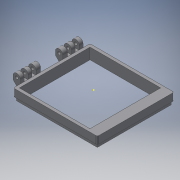
# Autodesk Inventor part: tampa extra
Saved by Autodesk Inventor 2019.4 (Build 234330000, 330)
## iProperties
Created: 2019-11-08
Part Number: tampa extra
Material: Genérico
Document SubType Name: Modeling
Designer: natha
Density: 1 g/cm^3
Appearance: Padrão
Author: natha
Autodesk Inventor part; units mm, degrees
ref_plane "YZ Plane" through (0, 0, 0) normal (1, 0, 0) x (0, 1, 0)
ref_plane "XZ Plane" through (0, 0, 0) normal (0, 1, 0) x (-1, 0, 0)
ref_plane "XY Plane" through (0, 0, 0) normal (0, 0, 1) x (1, 0, 0)
sketch "Esboço3" plane through (0, 0, 0) normal (0, 1, 0) x (-1, 0, 0)
  line L0 (-57, 52) -> (57, 52)
  line L1 (57, 52) -> (57, -52)
  line L2 (57, -52) -> (-57, -52)
  line L3 (-57, -52) -> (-57, 52)
  line L4 (-57, 52) -> (57, -52) construction
  line L5 (57, 52) -> (-57, -52) construction
  line L6 (-53, 48) -> (53, 48)
  line L7 (53, 48) -> (53, -48)
  line L8 (53, -48) -> (-53, -48)
  line L9 (-53, -48) -> (-53, 48)
  line L10 (-53, 48) -> (53, -48) construction
  line L11 (53, 48) -> (-53, -48) construction
  point P0 (0, 0)
  dimension "d9" = 104
  dimension "d10" = 114
  dimension "d11" = 106
  dimension "d12" = 96
  constraints: 24 end point, 4 midpoint, 4 parallel, 2 horizontal, 2 perpendicular
  measures "d9" distance of L0.end L1.end
  measures "d10" distance of L1.end L2.end
  measures "d11" distance of L7.end L8.end
  measures "d12" distance of L8.end L6.start
extrude "Extrusão2" add sketch "Esboço3" along normal blind 10
sketch "Esboço4" plane through (0, 0, 0) normal (0, -1, 0) x (1, 0, 0)
  line L0 (-53, -48) -> (53, -48) projected
  line L1 (-53, 48) -> (53, 48)
  line L2 (53, 48) -> (53, -48)
  line L3 (53, -48) -> (-53, -48)
  line L4 (-53, -48) -> (-53, 48)
  line L5 (-53, 48) -> (53, -48) construction
  line L6 (53, 48) -> (-53, -48) construction
  line L7 (-55, 50) -> (55, 50)
  line L8 (55, 50) -> (55, -50)
  line L9 (55, -50) -> (-55, -50)
  line L10 (-55, -50) -> (-55, 50)
  line L11 (-55, 50) -> (55, -50) construction
  line L12 (55, 50) -> (-55, -50) construction
  point P0 (0, 0)
  dimension "d15" = 100
  dimension "d16" = 96
  dimension "d17" = 110
  dimension "d18" = 106
  constraints: 24 end point, 4 midpoint, 4 parallel, 2 horizontal, 2 perpendicular
  measures "d15" distance of L7.end L8.end
  measures "d16" distance of L1.end L0.end
  measures "d17" distance of L8.end L9.end
  measures "d18" distance of L0.start L0.end
extrude "Extrusão3" add sketch "Esboço4" along normal blind 5
sketch "Esboço5" plane through (0, 10, 0) normal (0, 1, 0) x (1, 0, 0)
  line L0 (53, 48) -> (53, -48) projected
  line L1 (53, -48) -> (43, -48)
  line L2 (43, -48) -> (43, 48)
  line L3 (43, 48) -> (53, 48)
  line L4 (53, 48) -> (53, -48)
  point P0 (0, 0)
  dimension "d21" = 10
  constraints: 8 end point, 2 parallel, 1 horizontal, 1 perpendicular
  measures "d21" distance of L0.end L1.end
extrude "Extrusão4" add sketch "Esboço5" against normal blind 2
sketch "Esboço6" plane through (0, 8, 0) normal (0, -1, 0) x (1, 0, 0)
  line L0 (43, 48) -> (43, -48) projected
  line L1 (43, 48) -> (45, 48)
  line L2 (45, 48) -> (45, -48)
  line L3 (45, -48) -> (43, -48)
  line L4 (43, -48) -> (43, 48)
  point P0 (0, 0)
  dimension "d24" = 2
  constraints: 8 end point, 2 parallel, 1 horizontal, 1 perpendicular
  measures "d24" distance of L2.end L3.end
extrude "Extrusão5" add sketch "Esboço6" along normal blind 13
sketch "Esboço7" plane through (0, 10, 0) normal (0, 1, 0) x (1, 0, 0)
  point P0 (0, 0)
sketch "Esboço9" plane through (-57, 0, 52) normal (0, 0, 1) x (1, 0, 0)
  line L0 (114, 0) -> (0, 0) projected
  line L1 (0, 0) -> (-9.4142, 9.4142)
  line L2 (0, 0) -> (0, 10) projected
  line L3 (0, 10) -> (-10, 10) construction
  line L4 (0, 10) -> (0, 15.06) construction
  line L5 (0, 15.06) -> (-10, 15.06) construction
  arc A0 (0, 15.06) -> (-10, 15.06) centre (-5, 15.06) ccw
  line L6 (-10, 10.8284) -> (-10, 15.06)
  line L7 (0, 15.06) -> (0, 0)
  circle A1 centre (-5, 15.06) radius 2
  arc A2 (-10, 10.8284) -> (-9.4142, 9.4142) centre (-8, 10.8284) ccw
  point P0 (57, 0)
  dimension "d29" = 45
  dimension "d30" = 5.06
  dimension "d31" = 4
  dimension "d32" = 2
  constraints: 12 end point, 4 point on circle, 3 centre point, 3 tangent, 2 point on line, 2 vertical, 1 coincident, 1 collinear, 1 horizontal, 1 midpoint, 1 perpendicular
  measures "d29" angle of L1 L2
  measures "d30" distance of L2.end L4.end
  measures "d31" diameter of A1
  measures "d32" radius of A2
extrude "Extrusão6" add sketch "Esboço9" against normal blind 104
sketch "Esboço10" plane through (-67, 10.8284, 52) normal (-1, 0, 0) x (0, 0, 1)
  line L0 (-52, -10.8284) -> (-67, -10.8284) construction
  line L1 (-102, -10.8284) -> (-2, -10.8284) construction
  line L2 (-67, -10.8284) -> (-37, -10.8284) construction
  line L3 (-37, -10.8284) -> (-37, 9.2316) construction
  line L4 (0, 9.2316) -> (-104, 9.2316) construction
  line L5 (-67, 9.2316) -> (-37, 9.2316) construction
  line L6 (-67, -10.8284) -> (-67, 9.2316) construction
  line L7 (-104, 9.2316) -> (-94.5, 9.2316)
  line L8 (-94.5, 9.2316) -> (-94.5, -10.8284)
  line L9 (-94.5, -10.8284) -> (-104, -10.8284)
  line L10 (-104, -10.8284) -> (-104, 9.2316)
  line L11 (0, 9.2316) -> (-9.5, 9.2316)
  line L12 (-9.5, 9.2316) -> (-9.5, -10.8284)
  line L13 (-9.5, -10.8284) -> (0, -10.8284)
  line L14 (0, -10.8284) -> (0, 9.2316)
  line L15 (-67, 9.2316) -> (-37, 9.2316)
  line L16 (-37, 9.2316) -> (-37, -10.8284)
  line L17 (-37, -10.8284) -> (-67, -10.8284)
  line L18 (-67, -10.8284) -> (-67, 9.2316)
  line L19 (-94.5, 9.2316) -> (-89.5, 9.2316) construction
  line L20 (-9.5, 9.2316) -> (-14.5, 9.2316) construction
  line L21 (-89.5, 9.2316) -> (-83.9, 9.2316)
  line L22 (-83.9, 9.2316) -> (-83.9, -1.4142)
  line L23 (-83.9, -1.4142) -> (-89.5, -1.4142)
  line L24 (-89.5, -1.4142) -> (-89.5, 9.2316)
  line L25 (-14.5, 9.2316) -> (-20.1, 9.2316)
  line L26 (-20.1, 9.2316) -> (-20.1, -1.4142)
  line L27 (-20.1, -1.4142) -> (-14.5, -1.4142)
  line L28 (-14.5, -1.4142) -> (-14.5, 9.2316)
  line L29 (-83.9, 9.2316) -> (-78.9, 9.2316)
  line L30 (-20.1, 9.2316) -> (-25.1, 9.2316)
  line L31 (-78.9, 9.2316) -> (-73.3, 9.2316)
  line L32 (-73.3, 9.2316) -> (-73.3, -1.4142)
  line L33 (-73.3, -1.4142) -> (-78.9, -1.4142)
  line L34 (-78.9, -1.4142) -> (-78.9, 9.2316)
  line L35 (-25.1, 9.2316) -> (-30.7, 9.2316)
  line L36 (-30.7, 9.2316) -> (-30.7, -1.4142)
  line L37 (-30.7, -1.4142) -> (-25.1, -1.4142)
  line L38 (-25.1, -1.4142) -> (-25.1, 9.2316)
  dimension "d35" = 15
  dimension "d36" = 30
  dimension "d37" = 9.5
  dimension "d38" = 9.5
  dimension "d39" = 5
  dimension "d40" = 5
  dimension "d41" = 5.6
  dimension "d42" = 5.6
  dimension "d43" = 5
  dimension "d44" = 5
  dimension "d45" = 5.6
  dimension "d46" = 5.6
  constraints: 74 end point, 14 parallel, 10 point on line, 8 perpendicular, 7 horizontal, 1 collinear, 1 vertical
  measures "d35" distance of L0.start L0.end
  measures "d36" distance of L0.end L2.end
  measures "d37" distance of L8.end L9.end
  measures "d38" distance of L13.end L12.end
  measures "d39" distance of L7.end L19.end
  measures "d40" distance of L11.end L20.end
  measures "d41" distance of L22.end L23.end
  measures "d42" distance of L27.end L26.end
  measures "d43" distance of L21.end L29.end
  measures "d44" distance of L25.end L30.end
  measures "d45" distance of L32.end L33.end
  measures "d46" distance of L37.end L36.end
extrude "Extrusão7" cut sketch "Esboço10" against normal blind 10
fillet "Arredondamento1" radius 2 4 edges at (57, 5, 52) (57, 5, -52) (-57, 5, -52) (-57, 5, 52)
